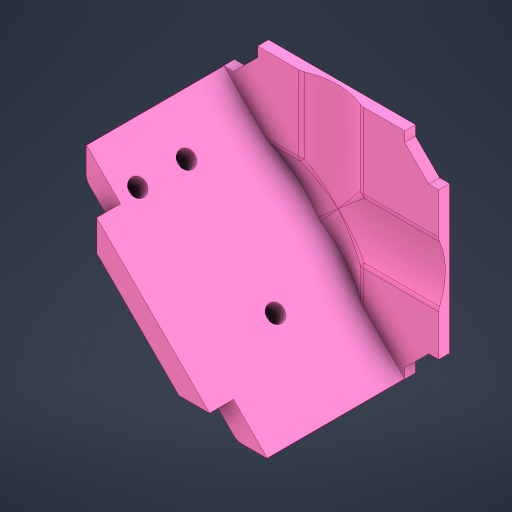
# Autodesk Inventor part: Mirror Base Horizontal
Saved by Autodesk Inventor 2023.4 (Build 274418000, 418)
## iProperties
Created: 2022-08-14
Part Number: Mirror Base Horizontal
Material: Generic
Document SubType Name: Modeling
Designer: xSibe
Density: 1 g/cm^3
Appearance: Plastic Pink
Author: xSibe
Autodesk Inventor part; units mm, degrees
sketch "Sketch1" plane through (0, 0, 0) normal (0, 0, 1) x (1, 0, 0)
  circle A0 centre (-10, 20.9) radius 1.875 projected
  circle A1 centre (-10, -20.9) radius 1.875 projected
  circle A2 centre (10, 20.9) radius 1.875 projected
  circle A3 centre (10, -20.9) radius 1.875 projected
  circle A4 centre (20.8, -14.4) radius 2.075 projected
  circle A5 centre (20.8, 14.4) radius 2.075 projected
  circle A6 centre (-20.8, 14.4) radius 2.075 projected
  circle A7 centre (-20.8, -14.4) radius 2.075 projected
  line L0 (16.9, -16.9) -> (-16.9, -16.9) projected
  line L1 (-16.9, -16.9) -> (-16.9, 16.9) projected
  line L2 (-16.9, 16.9) -> (16.9, 16.9) projected
  line L3 (16.9, 16.9) -> (16.9, -16.9) projected
  line L4 (-17.05, 24.9) -> (-17.05, 22.55) projected
  line L5 (-17.05, 22.55) -> (-22.55, 17.05) projected
  line L6 (-22.55, 17.05) -> (-24.9, 17.05) projected
  line L7 (-24.9, 17.05) -> (-24.9, -17.05) projected
  line L8 (-24.9, -17.05) -> (-22.55, -17.05) projected
  line L9 (-22.55, -17.05) -> (-17.05, -22.55) projected
  line L10 (-17.05, -22.55) -> (-17.05, -24.9) projected
  line L11 (-17.05, -24.9) -> (17.05, -24.9) projected
  line L12 (17.05, -24.9) -> (17.05, -22.55) projected
  line L13 (17.05, -22.55) -> (22.55, -17.05) projected
  line L14 (22.55, -17.05) -> (24.9, -17.05) projected
  line L15 (24.9, -17.05) -> (24.9, 17.05) projected
  line L16 (24.9, 17.05) -> (22.55, 17.05) projected
  line L17 (22.55, 17.05) -> (17.05, 22.55) projected
  line L18 (17.05, 22.55) -> (17.05, 24.9) projected
  line L19 (17.05, 24.9) -> (-17.05, 24.9) projected
  line L20 (-16.975, 24.825) -> (-16.975, 22.5189)
  line L21 (-16.975, 22.5189) -> (-22.5189, 16.975)
  line L22 (-22.5189, 16.975) -> (-24.825, 16.975)
  line L23 (-24.825, 16.975) -> (-24.825, -16.975)
  line L24 (-24.825, -16.975) -> (-22.5189, -16.975)
  line L25 (-22.5189, -16.975) -> (-16.975, -22.5189)
  line L26 (-16.975, -22.5189) -> (-16.975, -24.825)
  line L27 (-16.975, -24.825) -> (16.975, -24.825)
  line L28 (16.975, -24.825) -> (16.975, -22.5189)
  line L29 (16.975, -22.5189) -> (22.5189, -16.975)
  line L30 (22.5189, -16.975) -> (24.825, -16.975)
  line L31 (24.825, -16.975) -> (24.825, 16.975)
  line L32 (24.825, 16.975) -> (22.5189, 16.975)
  line L33 (22.5189, 16.975) -> (16.975, 22.5189)
  line L34 (16.975, 22.5189) -> (16.975, 24.825)
  line L35 (16.975, 24.825) -> (-16.975, 24.825)
  point P0 (0, 0)
  dimension "d0" = 0.075
  constraints: 32 end point, 15 other
  measures "d0" distance between parallel lines of L19 L35
ref_plane "Work Plane1" through (-24.9, -24.9, 7.7) normal (0, 0, 1) x (1, 0, 0)
extrude "Extrusion1" add sketch "Sketch1" along normal blind 2.5 from surface at 7.7 contours A0 | A1 | A2 | A3 | A4 | A5 | A6 | A7 | L0 L1 L2 L3 | L35 L34 L33 L32 L31 L30 L29 L28 L27 L26 L25 L24 L23 L22 L21 L20
sketch "Sketch2" plane through (-16.975, -24.825, 10.2) normal (0, 0, 1) x (1, 0, 0)
  line L0 (0, 47.3439) -> (0, 49.65) projected
  line L1 (-5.5439, 41.8) -> (0, 47.3439) projected
  line L2 (-7.85, 41.8) -> (-5.5439, 41.8) projected
  line L3 (-7.85, 7.85) -> (-7.85, 41.8) projected
  line L4 (-5.5439, 7.85) -> (-7.85, 7.85) projected
  line L5 (0, 2.3061) -> (-5.5439, 7.85) projected
  line L6 (0, 0) -> (0, 2.3061) projected
  line L7 (33.95, 0) -> (0, 0) projected
  line L8 (33.95, 2.3061) -> (33.95, 0) projected
  line L9 (39.4939, 7.85) -> (33.95, 2.3061) projected
  line L10 (41.8, 7.85) -> (39.4939, 7.85) projected
  line L11 (41.8, 41.8) -> (41.8, 7.85) projected
  line L12 (39.4939, 41.8) -> (41.8, 41.8) projected
  line L13 (33.95, 47.3439) -> (39.4939, 41.8) projected
  line L14 (33.95, 49.65) -> (33.95, 47.3439) projected
  line L15 (0, 49.65) -> (33.95, 49.65) projected
  line L16 (33.95, 49.65) -> (41.8, 49.65)
  line L17 (41.8, 49.65) -> (41.8, 41.8)
  line L18 (41.8, 41.8) -> (33.95, 41.8)
  line L19 (33.95, 41.8) -> (33.95, 49.65)
  line L20 (41.8, 49.65) -> (31.8, 49.65)
  line L21 (31.8, 49.65) -> (31.8, 44.65)
  line L22 (36.8, 39.65) -> (41.8, 39.65)
  line L23 (41.8, 39.65) -> (41.8, 49.65)
  line L24 (31.8, 44.65) -> (36.8, 39.65)
  line L25 (36.722, 5.078) -> (-2.772, 44.572)
  line L26 (34.9542, 3.3103) -> (-4.5397, 42.8042)
  line L27 (33.95, 0.0718) -> (-7.7782, 41.8)
  line L28 (26.9508, 0) -> (-7.85, 34.8008)
  line L29 (-7.85, 34.8008) -> (-0.075, 34.8008)
  line L30 (-0.075, 34.8008) -> (-0.075, 27.0258)
  line L31 (26.9508, 0) -> (26.9508, 7.775)
  line L32 (26.9508, 7.775) -> (19.1758, 7.775)
  line L33 (0.05, 33.9718) -> (0.05, 26.9008)
  line L34 (26.1218, 7.9) -> (19.0508, 7.9)
  point P0 (16.975, 24.825)
  point P1 (31.8, 39.65)
  point P2 (-4.5397, 42.8042)
  point P3 (34.9542, 3.3103)
  dimension "d3" = 10
  dimension "d4" = 10
  dimension "d5" = 5
  dimension "d6" = 5
  dimension "d7" = 2.5
  dimension "d8" = 3
  dimension "d9" = 5
  dimension "d35" = 7.775
  dimension "d36" = 7.775
  dimension "d37" = 0.125
  dimension "d38" = 0.125
  constraints: 38 end point, 12 point on line, 10 parallel, 4 perpendicular, 3 horizontal, 2 midpoint
  measures "d3" distance of L22.end point (31.8, 39.65)
  measures "d4" distance of point (31.8, 39.65) L20.end
  measures "d5" distance of L21.end point (31.8, 39.65)
  measures "d6" distance of L22.start point (31.8, 39.65)
  measures "d7" distance between parallel lines of L25 L26
  measures "d8" distance between parallel lines of L26 L27
  measures "d9" distance between parallel lines of L27 L28
  measures "d35" distance of L28.end L29.end
  measures "d36" distance of L28.start L31.end
  measures "d37" distance between parallel lines of L30 L33
  measures "d38" distance between parallel lines of L32 L34
extrude "Extrusion2" add sketch "Sketch2" along normal blind 31.75 contours L25 L9 L26 L1 | L27 L29 L3 L2 | L27 L30 L28 L29 | L8 L7 L31 L27 | L27 L33 L28 L30 | L31 L28 L32 L27 | L27 L34 L28 L33 | L32 L28 L34 L27
sketch "Sketch3" plane through (9.9758, -24.825, 10.2) normal (-0.7071068, -0.7071068, 0) x (0.7071068, -0.7071068, 0)
  line L0 (0, 0) -> (-49.2157, 0) projected
  line L1 (0, 0) -> (0, 31.75) projected
  line L2 (-49.2157, 31.75) -> (0, 31.75) projected
  line L3 (-49.2157, 0) -> (-49.2157, 31.75) projected
  line L4 (-49.2157, 15.875) -> (0, 15.875)
  line L5 (-5.2329, 4.625) -> (-43.9829, 4.625)
  line L6 (-43.9829, 4.625) -> (-43.9829, 27.125)
  line L7 (-43.9829, 27.125) -> (-5.2329, 27.125)
  line L8 (-5.2329, 27.125) -> (-5.2329, 4.625)
  line L9 (-5.2329, 4.625) -> (-43.9829, 27.125) construction
  line L10 (-43.9829, 4.625) -> (-5.2329, 27.125) construction
  circle A0 centre (-43.9829, 27.125) radius 1.9375
  circle A1 centre (-43.9829, 15.875) radius 1.9375
  line L11 (-24.6079, 15.875) -> (-5.2329, 15.875)
  circle A2 centre (-14.9204, 15.875) radius 1.9375
  line L12 (-52.5343, 0) -> (3.3186, 0) projected
  line L13 (-52.5343, 0) -> (-52.5343, 31.75) projected
  line L14 (3.3186, 31.75) -> (-52.5343, 31.75) projected
  line L15 (3.3186, 0) -> (3.3186, 31.75) projected
  line L16 (-0.75, 31) -> (-0.75, 0.75)
  line L17 (-0.75, 0.75) -> (-48.4657, 0.75)
  line L18 (-48.4657, 0.75) -> (-48.4657, 31)
  line L19 (-48.4657, 31) -> (-0.75, 31)
  circle A3 centre (-43.9829, 27.125) radius 2.5375
  circle A4 centre (-43.9829, 15.875) radius 2.5375
  circle A5 centre (-14.9204, 15.875) radius 2.5375
  point P0 (-24.6079, -10.2)
  point P1 (0, 31.75)
  point P2 (0, 0)
  point P3 (-49.2157, 31.75)
  point P4 (-0.75, 15.875)
  point P5 (-48.4657, 15.875)
  dimension "d12" = 38.75
  dimension "d13" = 22.5
  dimension "d14" = 3.875
  dimension "d15" = 3.875
  dimension "d16" = 3.875
  dimension "d21" = 0.75
  dimension "d22" = 5.075
  dimension "d23" = 5.075
  dimension "d24" = 5.075
  constraints: 24 end point, 8 midpoint, 6 centre point, 4 coincident, 2 parallel, 1 horizontal, 1 perpendicular, 3 other
  measures "d12" distance of L6.end L7.end
  measures "d13" distance of L5.end L6.end
  measures "d14" diameter of A0
  measures "d15" diameter of A1
  measures "d16" diameter of A2
  measures "d21" distance between parallel lines of L1 L16
  measures "d22" diameter of A3
  measures "d23" diameter of A4
  measures "d24" diameter of A5
extrude "Extrusion3" cut sketch "Sketch3" along normal blind 2.5 from surface at -10.5 contours L0 L3 L4 L18 L17 L16 L1 | L1 L14 L15 L12 | L12 L13 L14 L3 | L4 L16 L19 L18 L3 L2 L1
extrude "Extrusion4" cut sketch "Sketch3" against normal up to surface (5 mm away) contours A1 L6 L4 | L4 L6 A1 | A2 L4 | L4 A2 | L6 A1 L4 | L4 A1 L6 | A0 L6 L7 | L7 L6 A0
extrude "Extrusion5" cut sketch "Sketch3" against normal blind 1.5 from surface at -8 contours A4 L6 A1 L4 | L4 A1 L6 A4 | A5 L4 A2 | L4 A2 A5 | A1 L6 L4 | L4 L6 A1 | A4 L4 A1 L6 | L6 A1 L4 A4 | A2 L4 | L4 A2 | A3 L6 A0 L7 | L7 A0 L6 A3 | L6 A1 L4 | L4 A1 L6 | A0 L6 L7 | L7 L6 A0
extrude "Extrusion6" cut sketch "Sketch3" along normal blind 2.5 from surface at -10.5
sketch "Sketch4" plane through (0, 0, 0) normal (0, 1, 0) x (-1, 0, 0)
  line L0 (22.9, 0.025) -> (-22.9, 0.025) projected
  line L1 (22.9, 42.1) -> (22.9, 0.025) projected
  line L2 (22.9, 42.1) -> (17.05, 42.1) projected
  line L3 (17.05, 7.7) -> (17.05, 42.1) projected
  line L4 (-17.05, 7.7) -> (17.05, 7.7) projected
  line L5 (-17.05, 7.7) -> (-17.05, 42.1) projected
  line L6 (-17.05, 42.1) -> (-22.9, 42.1) projected
  line L7 (-22.9, 0.025) -> (-22.9, 42.1) projected
  circle A0 centre (19.9, 34.8) radius 2.0625 projected
  circle A1 centre (-19.9, 34.8) radius 2.0625 projected
  circle A2 centre (19.9, 15) radius 2.0625 projected
  circle A3 centre (-19.9, 15) radius 2.0625 projected
  circle A4 centre (10, 3.85) radius 1.5625 projected
  circle A5 centre (-10, 3.85) radius 1.5625 projected
  line L8 (-17.05, 24.9) -> (17.05, 24.9)
  circle A6 centre (0, 24.9) radius 16.25
  point P0 (0, 0)
  dimension "d27" = 32.5
  constraints: 3 midpoint, 2 end point, 1 centre point
  measures "d27" diameter of A6
ref_plane "Work Plane2" through (-22.9, 24.9, 0.025) normal (0, 1, 0) x (0, 0, 1)
extrude "Extrusion7" cut sketch "Sketch4" against normal up to surface from surface at 24.9 contours A6 L8 | L8 A6 surface through (16.975, -24.7532, 10.2) normal (0.7071068, 0.7071068, 0)
ref_plane "Work Plane3" through (0, 0, 0) normal (0.7071068, -0.7071068, 0) x (0, 0, -1)
mirror "Mirror1" about plane through (0, 0, 0) normal (0.7071068, -0.7071068, 0) of "Extrusion7"
extrude "Extrusion8" cut sketch "Sketch2" against normal up to surface (2.5 mm away) contours L28 L7 L6 L5 L4 L3
fillet "Fillet1" radius 2.5 12 edges at (9.9758, -24.825, 24.825) (-24.825, 9.9758, 24.825) (6.9262, 15.8756, 10.2) (15.8756, 6.9262, 10.2) (15.8756, -6.9262, 10.2) (6.9262, -10.8153, 10.2) (3.5488, 3.5488, 9.0422) (3.5488, -3.5488, 9.0422) (-1.9588, -1.9588, 8.7685) (-3.5488, 3.5488, 9.0422) (-6.9262, 15.8756, 10.2) (-10.8153, 6.9262, 10.2)
extrude "Extrusion9" add sketch "Sketch2" along normal blind 5.5 from surface at 31.75 contours L27 L34 L28 L33
equation "\"d6\" = d5"
body "Solid1"
